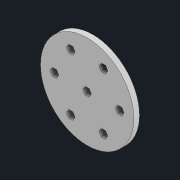
# Autodesk Inventor part: Input _Ring
Saved by Autodesk Inventor 2022 (Build 260153000, 153)
## iProperties
Created: 2022-01-11
Part Number: Input _Ring
Material: Generic
Document SubType Name: Modeling
Designer: divid
Density: 1 g/cm^3
Appearance: Default
Author: divid
Autodesk Inventor part; units mm, degrees
ref_plane "YZ Plane" through (0, 0, 0) normal (1, 0, 0) x (0, 1, 0)
ref_plane "XZ Plane" through (0, 0, 0) normal (0, 1, 0) x (-1, 0, 0)
ref_plane "XY Plane" through (0, 0, 0) normal (0, 0, 1) x (1, 0, 0)
sketch "Sketch1" plane through (0, 0, 0) normal (0, 0, 1) x (1, 0, 0)
  circle A0 centre (0, 0) radius 31.75
  dimension "d0" = 63.5
  constraints: 1 centre point, 1 coincident
  measures "d0" diameter of A0
extrude "Extrusion1" add sketch "Sketch1" along normal blind 3.81
sketch "Sketch2" plane through (0, 0, 3.81) normal (0, 0, 1) x (1, 0, 0)
  line L0 (-11.1125, 19.2474) -> (11.1125, 19.2474)
  line L1 (11.1125, 19.2474) -> (22.225, 0)
  line L2 (22.225, 0) -> (11.1125, -19.2474)
  line L3 (11.1125, -19.2474) -> (-11.1125, -19.2474)
  line L4 (-11.1125, -19.2474) -> (-22.225, 0)
  line L5 (-22.225, 0) -> (-11.1125, 19.2474)
  line L6 (-12.5559, 21.7474) -> (-9.6691, 21.7474)
  line L7 (-9.6691, 21.7474) -> (-8.2257, 19.2474)
  line L8 (-8.2257, 19.2474) -> (-9.6691, 16.7474)
  line L9 (-9.6691, 16.7474) -> (-12.5559, 16.7474)
  line L10 (-12.5559, 16.7474) -> (-13.9993, 19.2474)
  line L11 (-13.9993, 19.2474) -> (-12.5559, 21.7474)
  line L12 (-23.6684, -2.5) -> (-25.1118, 0)
  line L13 (-25.1118, 0) -> (-23.6684, 2.5)
  line L14 (-23.6684, 2.5) -> (-20.7816, 2.5)
  line L15 (-20.7816, 2.5) -> (-19.3382, 0)
  line L16 (-19.3382, 0) -> (-20.7816, -2.5)
  line L17 (-20.7816, -2.5) -> (-23.6684, -2.5)
  line L18 (-9.6691, -21.7474) -> (-12.5559, -21.7474)
  line L19 (-12.5559, -21.7474) -> (-13.9993, -19.2474)
  line L20 (-13.9993, -19.2474) -> (-12.5559, -16.7474)
  line L21 (-12.5559, -16.7474) -> (-9.6691, -16.7474)
  line L22 (-9.6691, -16.7474) -> (-8.2257, -19.2474)
  line L23 (-8.2257, -19.2474) -> (-9.6691, -21.7474)
  line L24 (13.9993, -19.2474) -> (12.5559, -21.7474)
  line L25 (12.5559, -21.7474) -> (9.6691, -21.7474)
  line L26 (9.6691, -21.7474) -> (8.2257, -19.2474)
  line L27 (8.2257, -19.2474) -> (9.6691, -16.7474)
  line L28 (9.6691, -16.7474) -> (12.5559, -16.7474)
  line L29 (12.5559, -16.7474) -> (13.9993, -19.2474)
  line L30 (23.6684, 2.5) -> (25.1118, 0)
  line L31 (25.1118, 0) -> (23.6684, -2.5)
  line L32 (23.6684, -2.5) -> (20.7816, -2.5)
  line L33 (20.7816, -2.5) -> (19.3382, 0)
  line L34 (19.3382, 0) -> (20.7816, 2.5)
  line L35 (20.7816, 2.5) -> (23.6684, 2.5)
  line L36 (9.6691, 21.7474) -> (12.5559, 21.7474)
  line L37 (12.5559, 21.7474) -> (13.9993, 19.2474)
  line L38 (13.9993, 19.2474) -> (12.5559, 16.7474)
  line L39 (12.5559, 16.7474) -> (9.6691, 16.7474)
  line L40 (9.6691, 16.7474) -> (8.2257, 19.2474)
  line L41 (8.2257, 19.2474) -> (9.6691, 21.7474)
  point P0 (0, 0)
  point P1 (0, 0)
  point P2 (0, 0)
  dimension "d15" = 5
  dimension "d18" = 360
  dimension "d20" = 22.225
  constraints: 84 end point, 3 coincident, 2 horizontal, 99 other
  measures "d15" distance between parallel lines of L9 L6
  measures "d20" distance of L0.start L0.end
extrude "Extrusion2" cut sketch "Sketch2" against normal blind 3.81 contours L5 L10 L11 L6 L7 L0 | L0 L8 L9 L5 | L41 L36 L37 L38 L1 L0 | L0 L1 L39 L40 | L15 L16 L4 L5 | L5 L4 L17 L12 L13 L14 | L35 L30 L31 L32 L2 L1 | L1 L2 L33 L34 | L21 L22 L3 L4 | L4 L3 L23 L18 L19 L20 | L29 L24 L25 L26 L3 L2 | L2 L3 L27 L28
sketch "Sketch3" plane through (0, 0, 3.81) normal (0, 0, 1) x (1, 0, 0)
  circle A0 centre (0, 0) radius 31.75 projected
  line L0 (-2.8868, 0) -> (-1.4434, 2.5)
  line L1 (-1.4434, 2.5) -> (1.4434, 2.5)
  line L2 (1.4434, 2.5) -> (2.8868, 0)
  line L3 (2.8868, 0) -> (1.4434, -2.5)
  line L4 (1.4434, -2.5) -> (-1.4434, -2.5)
  line L5 (-1.4434, -2.5) -> (-2.8868, 0)
  dimension "d14" = 5
  constraints: 12 end point, 1 coincident, 13 other
  measures "d14" distance between parallel lines of L4 L1
extrude "Extrusion3" cut sketch "Sketch3" against normal blind 3.81 contours L0 L1 L2 L3 L4 L5
body "Solid1"
